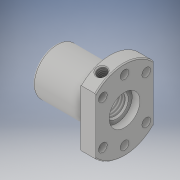
# Autodesk Inventor part: C-TBSE1204_n
Saved by Autodesk Inventor 2021 (Build 250183000, 183)
## iProperties
Created: 2023-01-12
Part Number: C-TBSE1204_n
Material: Generic
Catalog Web Link: www.cadenas.de
Description: C-TBSE1204, C-TBSE1205, C-TBSE1210, C-TBSB1204, C-TBSB1205, C-TBSB1210_nut-Economy Rolled Ball Screws - Thread Diameter 12, Lead 4/5/10 Precision Grade C7
Vendor: MISUMI
Document SubType Name: Modeling
Designer: psAdmin
Manufacturer: MISUMI
Mass: 16.7479 g
Surface Area: 71.1352 cm^2
Volume: 16.7479 cm^3
Density: 1 g/cm^3
Appearance: PSOLRGB-175-175-175
Category: PARTsolutions
Company: MISUMI
PSOL_IDENT_0: {$CADENAS_DATA/23d-libs/misumi/metric/09_ball_screws/c_tbse12/c_tbse12_nut.prj},242 {VTYP=3D},{NB=C-
PSOL_IDENT_1: TBSE1204_n},{LINA=C-TBSE1204},{NN=C-TBSE1204, C-TBSE1205, C-TBSE1210, C-TBSB1204, C-TBSB1205, C-TBSB
PSOL_IDENT_2: 1210_nut},{DATE=21.09.2022 00:19:55},{GEOMDATE=19.05.2021 06:54:52},{VERSION=},{LINEID=30},{WBVAR=TS
PSOL_IDENT_3: ,LEAD,ALT4},{WBNUMERIC=}  {NB=C-TBSE1204_n},{LINA=C-TBSE1204},{KT=DUMMY},{PN=C-TBSE1204},{TS=E},{TYP
PSOL_IDENT_4: E=C-TBSE},{AG=C7},{THRD=12},{LEAD=04},{A=35},{B=28.0},{T=8},{H=42},{C=32},{V=30},{ALT4=},{A1=7.6},{A
PSOL_IDENT_5: 2=8},{A3=0.9},{A4=7.9},{A5=10},{A6=24},{C1=0.5},{R=0.3},{B1=10},{B2=26},{B3=11},{B4=10},{B5=12},{B6=
PSOL_IDENT_6: 8},{M=6},{PITCH=1.0}
NB: C-TBSE1204_n
NN: C-TBSE1204, C-TBSE1205, C-TBSE1210, C-TBSB1204, C-TBSB1205, C-TBSB1210_nut
NT: Economy Rolled Ball Screws - Thread Diameter 12, Lead 4/5/10 Precision Grade C7
NBSYN: $PN._n
LINA: C-TBSE1204
CATALOG: Misumi
PN: C-TBSE1204
TS: EK Type
TYPE: C-TBSE
AG: C7
THRD: 12
LEAD: 04
ALT4: w/o RLC (Nut Direction)
SUPPLIER: MISUMI
ARTICLENO: C-TBSE1204_n
BOMINFO: C-TBSE1204
CREATOR: CADENAS GmbH
Title: C-TBSE1204
Author: Cadenas PARTsolutions
Comments: Economy Rolled Ball Screws - Thread Diameter 12, Lead 4/5/10 Precision Grade C7
Autodesk Inventor part; units mm, degrees
ref_plane "YZ Plane" through (0, 0, 0) normal (1, 0, 0) x (0, 1, 0)
ref_plane "XZ Plane" through (0, 0, 0) normal (0, 1, 0) x (-1, 0, 0)
ref_plane "XY Plane" through (0, 0, 0) normal (0, 0, 1) x (1, 0, 0)
sketch "Sketch_1" plane through (0, 0, 0) normal (0, 0, 1) x (1, 0, 0)
  line L0 (28, 0) -> (0, 0)
  line L1 (0, 0) -> (0, 11)
  arc A0 (1, 12) -> (0, 11) centre (1, 11) ccw
  line L2 (1, 12) -> (28, 12)
  line L3 (28, 12) -> (28, 0)
  line L4 (28, 0) -> (0, 0)
  constraints: 10 end point, 2 point on circle, 1 centre point
revolve "Revolution1" add sketch "Sketch_1" angle 360 about axis through (28, 0, 0) along (1, 0, 0)
sketch "_____2" plane through (0, 0, 0) normal (0, 0, 1) x (1, 0, 0)
  line L0 (36, 0) -> (28, 0)
  line L1 (28, 0) -> (28, 20.5)
  arc A0 (28.5, 21) -> (28, 20.5) centre (28.5, 20.5) ccw
  line L2 (28.5, 21) -> (35.5, 21)
  arc A1 (36, 20.5) -> (35.5, 21) centre (35.5, 20.5) ccw
  line L3 (36, 20.5) -> (36, 0)
  line L4 (36, 0) -> (28, 0)
  constraints: 10 end point, 4 point on circle, 2 centre point
revolve "Revolution2" add sketch "_____2" angle 360 about axis through (36, 0, 0) along (1, 0, 0)
sketch "_____3" plane through (28, 0, 0) normal (1, 0, 0) x (0, 0, -1)
  line L0 (-30, -21) -> (-15, -21)
  line L1 (-15, -21) -> (-15, 26)
  line L2 (-15, 26) -> (15, 26)
  line L3 (15, 26) -> (15, -21)
  line L4 (15, -21) -> (30, -21)
  line L5 (30, -21) -> (30, 31)
  line L6 (30, 31) -> (-30, 31)
  line L7 (-30, 31) -> (-30, -21)
  constraints: 16 end point
extrude "Extrusion1" cut sketch "_____3" along normal blind 8
sketch "Sketch4" plane through (28, -13.9732, -15) normal (-1, 0, 0) x (0, 0, 1)
  point P0 (15, 29.9732)
hole "Hole1" at (28, 16, 0) direction (1, 0, 0) diameter 4.5 depth 8
pattern_circular "Circular Pattern1" count 8 over 360 about axis through (28, 0, 0) along (1, 0, 0) of "Hole1" skipped copies 3 7
sketch "_____6" plane through (32, 0, 0) normal (1, 0, 0) x (0, 0, -1)
  line L0 (-8.0364, 19.4015) -> (0, 0)
  line L1 (0, 0) -> (-2.2714, -0.9408)
  line L2 (-2.2714, -0.9408) -> (-10.1005, 17.9604)
  line L3 (-10.1005, 17.9604) -> (-10.808, 18.2534)
  line L4 (-10.808, 18.2534) -> (-8.0364, 19.4015)
  line L5 (-8.0364, 19.4015) -> (0, 0)
  constraints: 12 end point
revolve "Revolution3" cut sketch "_____6" angle 360 about axis through (32, 19.4015, 8.0364) along (0, 0.9238795, 0.3826834)
thread "Thread1" size "M6x1" class "6H" standard "ISO Metric profile" length 7.4585
sketch "_____7" plane through (0, 0, 0) normal (0, 0, 1) x (1, 0, 0)
  line L0 (4, 0) -> (0, 0)
  line L1 (0, 0) -> (0, 8)
  line L2 (0, 8) -> (4, 8)
  line L3 (4, 8) -> (4, 0)
  line L4 (4, 0) -> (0, 0)
  constraints: 10 end point
revolve "Revolution4" cut sketch "_____7" angle 360 about axis through (4, 0, 0) along (1, 0, 0)
sketch "Sketch7" plane through (36, -13.9732, -15) normal (1, 0, 0) x (0, 0, -1)
  point P0 (-15, 13.9732)
hole "Hole2" at (36, 0, 0) direction (-1, 0, 0) diameter 16 depth 4
sketch "Sketch_8" plane through (0, 0, 0) normal (0, 0, 1) x (1, 0, 0)
  line L0 (32, 0) -> (4, 0)
  line L1 (4, 0) -> (4, 6)
  line L2 (4, 6) -> (4.812, 5.188)
  line L3 (4.812, 5.188) -> (31.188, 5.188)
  line L4 (31.188, 5.188) -> (32, 6)
  line L5 (32, 6) -> (32, 0)
  line L6 (32, 0) -> (4, 0)
  constraints: 14 end point
revolve "Revolution5" cut sketch "Sketch_8" angle 360 about axis through (32, 0, 0) along (1, 0, 0)
thread "Thread2" size "M12x1.5" class "6H" standard "ISO Metric profile" full length
ref_plane "NUT_XY" through (18, 0, 0) normal (1, 0, 0) x (0, 0, -1)
ref_plane "NUT_YZ" through (18, 0, 0) normal (0, 0, -1) x (0, 1, 0)
ref_plane "NUT_ZX" through (18, 0, 0) normal (0, 1, 0) x (1, 0, 0)
ref_plane "NUT2_XY" through (18, 0, 0) normal (1, 0, 0) x (0, 0, -1)
ref_plane "NUT2_YZ" through (18, 0, 0) normal (0, 0, -1) x (0, 1, 0)
ref_plane "NUT2_ZX" through (18, 0, 0) normal (0, 1, 0) x (1, 0, 0)
body "Solid1"
